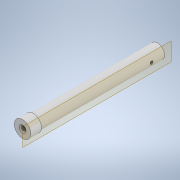
# Autodesk Inventor part: Glashalter
Saved by Autodesk Inventor 2021.3 (Build 253353000, 353)
## iProperties
Created: 2021-10-18
Part Number: Glashalter
Material: Generisch
Document SubType Name: Modeling
Designer: bhelg
Density: 1 g/cm^3
Appearance: Vorgabe
Author: bhelg
Autodesk Inventor part; units mm, degrees
note: some values were not read from the file. Chosen so that the rebuilt part matches the saved one: direction of "Bohrung4".
ref_plane "XZ Plane" through (0, 0, 0) normal (0, 1, 0) x (-1, 0, 0)
ref_plane "XY Plane" through (0, 0, 0) normal (0, 0, 1) x (1, 0, 0)
sketch "Skizze1" plane through (0, 0, 0) normal (0, 1, 0) x (-1, 0, 0)
  line L0 (0, 0) -> (7, 0)
  line L1 (7, 0) -> (7, -9)
  line L2 (7, -9) -> (6, -9)
  line L3 (6, -9) -> (6, -114)
  line L4 (6, -114) -> (0, -114)
  line L5 (0, -114) -> (0, 0)
  dimension "d0" = 7
  dimension "d1" = 6
  dimension "d2" = 9
  dimension "d3" = 105
  constraints: 12 end point, 4 perpendicular, 2 horizontal
  measures "d0" distance of L0.start L0.end
  measures "d1" distance from line of L0.start L3
  measures "d2" distance between parallel lines of L0 L2
  measures "d3" distance of L2.end L3.end
revolve "Umdrehung2" add sketch "Skizze1" angle 360 about axis through (0, 0, -114) along (0, 0, 1)
sketch "Skizze3" plane through (0, 0, -114) normal (0, 0, -1) x (-1, 0, 0)
  point P0 (0, 0)
  point P1 (0, 0)
  constraints: 1 coincident
hole "Bohrung2" at (0, 0, -114) direction (0, 0, 1) diameter 6.647 depth 8 tip angle 118 thread size "M8x1.25" class "6H" standard "ISO Metric profile"
sketch "Skizze4" plane through (0, 0, 0) normal (0, 0, 1) x (1, 0, 0)
  circle A0 centre (0, 0) radius 3.3235 projected
  point P0 (0, 0)
  constraints: 1 coincident
hole "Bohrung3" at (0, 0, 0) direction (0, 0, -1) diameter 4 end through all
chamfer "Fase2" distance 1 angle 45 1 edges at (0, 2, 0)
ref_plane "Arbeitsebene2" through (6, 0, 0) normal (1, 0, 0) x (0, 1, 0)
sketch "Skizze5" plane through (6, 0, 0) normal (1, 0, 0) x (0, 1, 0)
  line L0 (-6, -114) -> (6, -114) projected
  line L1 (0, 0) -> (0, -114)
  point P0 (0, -103)
  dimension "d39" = 11
  constraints: 2 end point, 1 midpoint, 1 point on line
  measures "d39" distance from line of point (0, -103) L0
hole "Bohrung4" at (6, 0, -103) direction (-1, 0, 0) diameter 2.459 end up to surface thread size "M3x0.5" class "6H" standard "ISO Metric profile"
